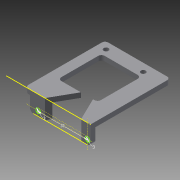
# Autodesk Inventor part: bart z endstop bracket v3
Saved by Autodesk Inventor 2014 SP1 (Build 180222100, 222)
## iProperties
Created: 2015-06-08
Part Number: bart z endstop bracket v3
Material: Generic
Document SubType Name: Modeling
Designer: Mon
Density: 1 g/cm^3
Appearance: Default
Author: Mon
Autodesk Inventor part; units mm, degrees
ref_plane "YZ Plane" through (0, 0, 0) normal (1, 0, 0) x (0, 1, 0)
ref_plane "XZ Plane" through (0, 0, 0) normal (0, 1, 0) x (-1, 0, 0)
ref_plane "XY Plane" through (0, 0, 0) normal (0, 0, 1) x (1, 0, 0)
sketch "Sketch1" plane through (0, 0, 0) normal (0, 0, 1) x (1, 0, 0)
  line L0 (0, 0) -> (53, 0)
  line L1 (53, 0) -> (53, -50)
  line L2 (53, -50) -> (0, -50)
  line L3 (0, -50) -> (0, 0)
  line L4 (41, 0) -> (41, 6.0159) construction
  line L5 (41, 6.0159) -> (41, -25.0024) construction
  circle A0 centre (41, -5) radius 1.5
  line L6 (41, 3.3654) -> (9, 3.3654) construction
  line L7 (9, 3.3654) -> (9, -23.8563) construction
  line L8 (41, -5) -> (7.1054, -5) construction
  circle A1 centre (9, -5) radius 1.5
  dimension "d0" = 53
  dimension "d1" = 50
  dimension "d2" = 3
  dimension "d3" = 32
  dimension "d4" = 3
  constraints: 18 end point, 5 point on line, 4 parallel, 3 perpendicular, 2 centre point, 1 collinear, 1 horizontal
  measures "d0" distance of L1.end L2.end
  measures "d1" distance of L0.end L1.end
  measures "d2" diameter of A0
  measures "d3" distance of L6.start L6.end
  measures "d4" diameter of A1
extrude "Extrusion1" add sketch "Sketch1" along normal blind 3
sketch "Sketch2" plane through (0, 0, 3) normal (0, 0, 1) x (1, 0, 0)
  line L0 (53, -50) -> (15, -50)
  line L1 (15, -50) -> (15, -47)
  line L2 (15, -47) -> (53, -47)
  line L3 (53, -47) -> (53, -50)
  dimension "d7" = 38
  dimension "d8" = 3
  constraints: 8 end point, 2 parallel, 1 horizontal, 1 perpendicular
  measures "d7" distance of L1.end L2.end
  measures "d8" distance of L0.end L1.end
extrude "Extrusion2" add sketch "Sketch2" against normal blind 12
fillet "Fillet3" radius 2 1 edges at (53, -48.5, -9)
fillet "Fillet6" radius 2 1 edges at (15, -48.5, -9)
sketch "Sketch5" plane through (0, 0, 3) normal (0, 0, 1) x (1, 0, 0)
  line L0 (18.1552, -8.3715) -> (42.9873, -8.3715)
  line L1 (42.9873, -8.3715) -> (42.9873, -35.5989)
  line L2 (42.9873, -35.5989) -> (18.1552, -35.5989)
  line L3 (18.1552, -35.5989) -> (18.1552, -8.3715)
  constraints: 8 end point, 2 parallel, 1 horizontal, 1 perpendicular
extrude "Extrusion4" cut sketch "Sketch5" against normal through all
fillet "Fillet8" radius 2 1 edges at (18.1552, -8.3715, 1.5)
fillet "Fillet9" radius 2 1 edges at (42.9873, -8.3715, 1.5)
fillet "Fillet10" radius 2 1 edges at (18.1552, -35.5989, 1.5)
fillet "Fillet12" radius 2 1 edges at (42.9873, -35.5989, 1.5)
fillet "Fillet13" radius 2 1 edges at (0, 0, 1.5)
fillet "Fillet14" radius 2 1 edges at (53, 0, 1.5)
hole "Hole3" at (17.1081, -4.4429, 3) direction (0, 0, -1) diameter 3 end through all
sketch "Sketch6" plane through (0, -50, 3) normal (0, -1, 0) x (1, 0, 0)
  line L0 (51, -12) -> (17, -12) projected
  line L1 (0, 0) -> (53, 0) projected
  line L2 (53, 0) -> (51, 0) construction
  line L3 (51, 2) -> (51, -15) construction
  line L4 (54, -9) -> (12.4146, -9) construction
  line L5 (51, -7.4819) -> (20, -7.4819) construction
  line L6 (20, -7.4819) -> (20, -11) construction
  circle A0 centre (20, -9) radius 1.5
  circle A1 centre (51, -9) radius 1.5
  dimension "d60" = 31
  dimension "d61" = 3
  dimension "d64" = 3
  constraints: 10 end point, 6 point on line, 2 centre point, 2 perpendicular, 1 parallel
  measures "d60" distance of L5.start L5.end
  measures "d61" diameter of A0
  measures "d64" diameter of A1
extrude "Extrusion5" cut sketch "Sketch6" against normal through all contours A0
extrude "Extrusion6" cut sketch "Sketch6" against normal through all contours A1
sketch "Sketch7" plane through (0, 0, 3) normal (0, 0, 1) x (1, 0, 0)
  line L0 (40.9873, -35.5989) -> (20.1552, -35.5989) projected
  line L1 (0, -50) -> (53, -50) projected
  line L2 (32.5151, -35.5989) -> (24.407, -50)
  line L3 (40.0869, -35.5989) -> (47.0869, -50)
  point P0 (0, 0)
  constraints: 4 end point, 4 point on line
extrude "Extrusion7" cut sketch "Sketch7" against normal through all
sketch "Sketch8" plane through (0, 0, 3) normal (0, 0, 1) x (1, 0, 0)
  line L0 (0, -50) -> (24.407, -50) projected
  circle A0 centre (9, -5) radius 1.5 projected
  line L1 (0, 0) -> (12, 0)
  line L2 (12, 0) -> (12, -50)
  line L3 (12, -50) -> (0, -50)
  line L4 (0, -50) -> (0, 0)
  constraints: 8 end point, 2 parallel, 1 horizontal, 1 perpendicular, 1 point on line
extrude "Extrusion8" cut sketch "Sketch8" against normal through all
fillet "Fillet15" radius 2 1 edges at (12, -50, 1.5)
fillet "Fillet16" radius 2 1 edges at (12, 0, 1.5)
body "Solid1"
